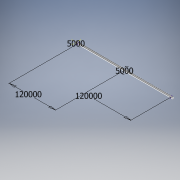
# Autodesk Inventor part: Fuel Distributor
Saved by Autodesk Inventor 2017.2 (Build 212233000, 233)
## iProperties
Created: 2017-03-31
Part Number: Fuel Distributor
Material: Aluminum 6061
Document SubType Name: Modeling
Designer: haden
Density: 2.7 g/cm^3
Appearance: Aluminum - Flat
Author: haden
Autodesk Inventor part; units mm, degrees
ref_plane "YZ Plane" through (0, 0, 0) normal (1, 0, 0) x (0, 1, 0)
ref_plane "XZ Plane" through (0, 0, 0) normal (0, 1, 0) x (-1, 0, 0)
ref_plane "XY Plane" through (0, 0, 0) normal (0, 0, 1) x (1, 0, 0)
sketch "Sketch1" plane through (0, 0, 0) normal (1, 0, 0) x (0, 1, 0)
  circle A0 centre (0, 0) radius 2500
  dimension "d0" = 5000
  constraints: 1 centre point, 1 coincident
  measures "d0" diameter of A0
extrude "Extrusion1" add sketch "Sketch1" along normal blind 250000
sketch "Sketch2" plane through (0, 0, 0) normal (0, 0, 1) x (1, 0, 0)
  line L0 (250000, -2500) -> (250000, 2500) projected
  circle A0 centre (5000, 0) radius 500
  circle A1 centre (125000, 0) radius 500
  circle A2 centre (245000, 0) radius 500
  point P0 (0, 0)
  dimension "d6" = 1000
  dimension "d7" = 120000
  dimension "d8" = 120000
  dimension "d9" = 5000
  constraints: 3 centre point, 3 horizontal alignment, 2 equal radius
  measures "d6" diameter of A0
  measures "d7" distance of A1.centre A2.centre
  measures "d8" distance of A0.centre A1.centre
  measures "d9" distance from line of A2.centre L0
extrude "Extrusion2" cut sketch "Sketch2" along normal through all both and the other way through all
sketch "Sketch3" plane through (0, 0, 0) normal (-1, 0, 0) x (0, 0, 1)
  line L0 (-2500, 2500) -> (2500, 2500)
  line L1 (2500, 2500) -> (2500, -2500)
  line L2 (2500, -2500) -> (-2500, -2500)
  line L3 (-2500, -2500) -> (-2500, 2500)
  point P0 (0, 0)
  dimension "d12" = 5000
  dimension "d13" = 2500
  dimension "d14" = 2500
  constraints: 8 end point, 2 parallel, 2 perpendicular, 1 horizontal
  measures "d12" distance of L0.start L0.end
  measures "d13" distance from line of point (0, 0) L3
  measures "d14" distance from line of L0 point (0, 0)
extrude "Extrusion3" add sketch "Sketch3" along normal blind 1000
sketch "Sketch4" plane through (0, 0, 0) normal (0, -1, 0) x (1, 0, 0)
  circle A0 centre (245000, 0) radius 2500
  circle A1 centre (125000, 0) radius 2500
  circle A2 centre (5000, 0) radius 2500
  point P0 (0, 0)
  dimension "d17" = 5000
  dimension "d18" = 120000
  dimension "d19" = 120000
  dimension "d20" = 5000
  constraints: 3 centre point, 3 horizontal alignment, 2 equal radius
  measures "d17" diameter of A1
  measures "d18" distance of A1.centre A0.centre
  measures "d19" distance of A2.centre A1.centre
  measures "d20" distance of point (0, 0) A2.centre
extrude "Extrusion4" add sketch "Sketch4" along normal mid plane 200000
body "Solid1"
